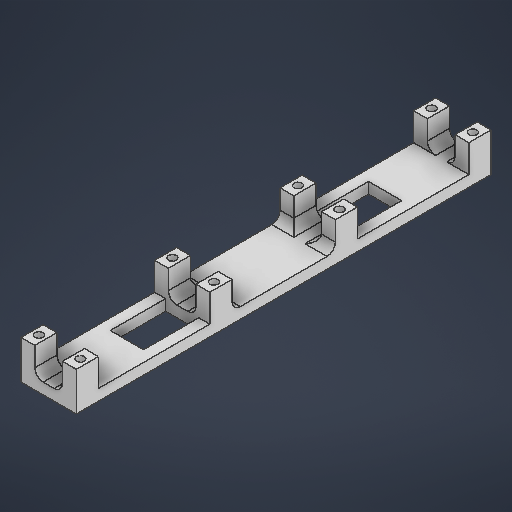
# Autodesk Inventor part: support_2_servos
Saved by Autodesk Inventor 2026.1 (Build 301233000, 233)
## iProperties
Created: 2025-10-11
Part Number: support_2_servos
Material: Generic
Document SubType Name: Modeling
Designer: emanuel
Density: 1 g/cm^3
Appearance: Default
Author: emanuel
Autodesk Inventor part; units mm, degrees
ref_plane "YZ Plane" through (0, 0, 0) normal (1, 0, 0) x (0, 1, 0)
ref_plane "XZ Plane" through (0, 0, 0) normal (0, 1, 0) x (-1, 0, 0)
ref_plane "XY Plane" through (0, 0, 0) normal (0, 0, 1) x (1, 0, 0)
sketch "Sketch1" plane through (0, 0, 0) normal (0, 1, 0) x (-1, 0, 0)
  line L0 (0, 0) -> (20, 0)
  line L1 (20, 0) -> (20, -150)
  line L2 (20, -150) -> (0, -150)
  line L3 (0, -150) -> (0, 0)
  dimension "d0" = 20
  dimension "d1" = 150
  constraints: 8 end point, 2 parallel, 1 horizontal, 1 perpendicular
  measures "d0" distance of L1.end L2.end
  measures "d1" distance of L0.end L1.end
extrude "Extrusion1" add sketch "Sketch1" along normal blind 4
sketch "Sketch2" plane through (0, 4, 0) normal (0, 1, 0) x (1, 0, 0)
  line L0 (-20, 0) -> (0, 0) projected
  line L1 (0, 0) -> (0, 150) projected
  line L2 (-20, 0) -> (0, 0)
  line L3 (0, 0) -> (0, 8)
  line L4 (0, 8) -> (-20, 8)
  line L5 (-20, 8) -> (-20, 0)
  line L6 (-20, 8) -> (0, 8)
  line L7 (0, 8) -> (0, 48.3)
  line L8 (0, 48.3) -> (-20, 48.3)
  line L9 (-20, 48.3) -> (-20, 8)
  line L10 (-20, 48.3) -> (0, 48.3)
  line L11 (0, 48.3) -> (0, 56.3)
  line L12 (0, 56.3) -> (-20, 56.3)
  line L13 (-20, 56.3) -> (-20, 48.3)
  line L14 (-20, 150) -> (-20, 0) projected
  line L15 (-20, 150) -> (0, 150)
  line L16 (0, 150) -> (0, 142)
  line L17 (0, 142) -> (-20, 142)
  line L18 (-20, 142) -> (-20, 150)
  line L19 (-20, 142) -> (0, 142)
  line L20 (0, 142) -> (0, 101.7)
  line L21 (0, 101.7) -> (-20, 101.7)
  line L22 (-20, 101.7) -> (-20, 142)
  line L23 (-20, 101.7) -> (0, 101.7)
  line L24 (0, 101.7) -> (0, 93.7)
  line L25 (0, 93.7) -> (-20, 93.7)
  line L26 (-20, 93.7) -> (-20, 101.7)
  line L27 (-20, 0) -> (-15, 0)
  line L28 (-15, 0) -> (-15, 8)
  line L29 (-15, 8) -> (-20, 8)
  line L30 (-20, 8) -> (-20, 0)
  line L31 (0, 8) -> (-5, 8)
  line L32 (-5, 8) -> (-5, 0)
  line L33 (-5, 0) -> (0, 0)
  line L34 (0, 0) -> (0, 8)
  line L35 (-20, 48.3) -> (-15, 48.3)
  line L36 (-15, 48.3) -> (-15, 56.3)
  line L37 (-15, 56.3) -> (-20, 56.3)
  line L38 (-20, 56.3) -> (-20, 48.3)
  line L39 (0, 48.3) -> (-5, 48.3)
  line L40 (-5, 48.3) -> (-5, 56.3)
  line L41 (-5, 56.3) -> (0, 56.3)
  line L42 (0, 56.3) -> (0, 48.3)
  line L43 (-20, 93.7) -> (-15, 93.7)
  line L44 (-15, 93.7) -> (-15, 101.7)
  line L45 (-15, 101.7) -> (-20, 101.7)
  line L46 (-20, 101.7) -> (-20, 93.7)
  line L47 (0, 93.7) -> (-5, 93.7)
  line L48 (-5, 93.7) -> (-5, 101.7)
  line L49 (-5, 101.7) -> (0, 101.7)
  line L50 (0, 101.7) -> (0, 93.7)
  line L51 (-20, 142) -> (-15, 142)
  line L52 (-15, 142) -> (-15, 150)
  line L53 (-15, 150) -> (-20, 150)
  line L54 (-20, 150) -> (-20, 142)
  line L55 (0, 142) -> (-5, 142)
  line L56 (-5, 142) -> (-5, 150)
  line L57 (-5, 150) -> (0, 150)
  line L58 (0, 150) -> (0, 142)
  point P0 (0, 142)
  point P1 (-20, 142)
  point P2 (-15, 93.7)
  point P3 (-15, 101.7)
  point P4 (-20, 101.7)
  point P5 (-20, 93.7)
  dimension "d4" = 8
  dimension "d5" = 40.3
  dimension "d6" = 8
  dimension "d7" = 20
  dimension "d8" = 8
  dimension "d9" = 40.3
  dimension "d10" = 8
  dimension "d11" = 5
  dimension "d12" = 5
  dimension "d13" = 8
  dimension "d14" = 5
  dimension "d15" = 5
  dimension "d16" = 5
  dimension "d17" = 5
  dimension "d18" = 5
  dimension "d19" = 5
  constraints: 112 end point, 28 parallel, 14 horizontal, 14 perpendicular, 12 point on line
  measures "d4" distance of L3.end L2.end
  measures "d5" distance of L7.end L6.end
  measures "d6" distance of L11.end L10.end
  measures "d7" distance of L16.end L17.end
  measures "d8" distance of L15.end L16.end
  measures "d9" distance of L19.end L20.end
  measures "d10" distance of L23.end L24.end
  measures "d11" distance of L29.end L28.end
  measures "d12" distance of L33.end L32.end
  measures "d13" distance of L32.end L31.end
  measures "d14" distance of L37.end L36.end
  measures "d15" distance of L40.end L41.end
  measures "d16" distance of L45.end L44.end
  measures "d17" distance of L48.end L49.end
  measures "d18" distance of L53.end L52.end
  measures "d19" distance of L56.end L57.end
extrude "Extrusion2" add sketch "Sketch2" along normal blind 10 contours L5 L4 L28 L0 | L32 L4 L1 L0 | L13 L12 L36 L8 | L40 L12 L1 L8 | L14 L21 L44 L25 | L14 L15 L52 L17 | L48 L21 L1 L25 | L56 L15 L1 L17
sketch "Sketch3" plane through (0, 14, 0) normal (0, 1, 0) x (1, 0, 0)
  line L0 (-20, 150) -> (-20, 0) projected
  line L1 (-20, 0) -> (-17.5, 0)
  line L2 (-17.5, 0) -> (-17.5, 4)
  line L3 (-17.5, 4) -> (-20, 4)
  line L4 (-20, 4) -> (-20, 0)
  line L5 (0, 0) -> (0, 150) projected
  line L6 (0, 0) -> (-2.5, 0)
  line L7 (-2.5, 0) -> (-2.5, 4)
  line L8 (-2.5, 4) -> (0, 4)
  line L9 (0, 4) -> (0, 0)
  line L10 (-15, 56.3) -> (-20, 56.3) projected
  line L11 (-20, 56.3) -> (-17.5, 56.3)
  line L12 (-17.5, 56.3) -> (-17.5, 52.3)
  line L13 (-17.5, 52.3) -> (-20, 52.3)
  line L14 (-20, 52.3) -> (-20, 56.3)
  line L15 (-5, 56.3) -> (0, 56.3) projected
  line L16 (-5, 56.3) -> (-2.5, 56.3)
  line L17 (-2.5, 56.3) -> (-2.5, 52.3)
  line L18 (-2.5, 52.3) -> (-5, 52.3)
  line L19 (-5, 52.3) -> (-5, 56.3)
  line L20 (-20, 150) -> (-17.5, 150)
  line L21 (-17.5, 150) -> (-17.5, 146)
  line L22 (-17.5, 146) -> (-20, 146)
  line L23 (-20, 146) -> (-20, 150)
  line L24 (-5, 150) -> (-2.5, 150)
  line L25 (-2.5, 150) -> (-2.5, 146)
  line L26 (-2.5, 146) -> (-5, 146)
  line L27 (-5, 146) -> (-5, 150)
  line L28 (-20, 101.7) -> (-15, 101.7) projected
  line L29 (-15, 101.7) -> (-17.5, 101.7)
  line L30 (-17.5, 101.7) -> (-17.5, 97.7)
  line L31 (-17.5, 97.7) -> (-15, 97.7)
  line L32 (-15, 97.7) -> (-15, 101.7)
  line L33 (-5, 101.7) -> (-2.5, 101.7)
  line L34 (-2.5, 101.7) -> (-2.5, 97.7)
  line L35 (-2.5, 97.7) -> (-5, 97.7)
  line L36 (-5, 97.7) -> (-5, 101.7)
  circle A0 centre (-17.5, 97.7) radius 1.5
  circle A1 centre (-2.5, 97.7) radius 1.5
  circle A2 centre (-17.5, 146) radius 1.5
  circle A3 centre (-2.5, 146) radius 1.5
  circle A4 centre (-17.5, 52.3) radius 1.5
  circle A5 centre (-2.5, 52.3) radius 1.5
  circle A6 centre (-17.5, 4) radius 1.5
  circle A7 centre (-2.5, 4) radius 1.5
  dimension "d22" = 2.5
  dimension "d23" = 4
  dimension "d24" = 2.5
  dimension "d25" = 4
  dimension "d26" = 2.5
  dimension "d27" = 4
  dimension "d28" = 2.5
  dimension "d29" = 4
  dimension "d30" = 2.5
  dimension "d31" = 4
  dimension "d32" = 2.5
  dimension "d33" = 4
  dimension "d34" = 2.5
  dimension "d35" = 4
  dimension "d36" = 2.5
  dimension "d37" = 4
  dimension "d38" = 3
  dimension "d39" = 3
  dimension "d40" = 3
  dimension "d41" = 3
  dimension "d42" = 3
  dimension "d43" = 3
  dimension "d44" = 3
  dimension "d45" = 3
  constraints: 64 end point, 16 parallel, 8 centre point, 8 coincident, 8 horizontal, 8 perpendicular, 4 point on line
  measures "d22" distance of L3.end L2.end
  measures "d23" distance of L2.end L1.end
  measures "d24" distance of L7.end L8.end
  measures "d25" distance of L6.end L7.end
  measures "d26" distance of L12.end L13.end
  measures "d27" distance of L11.end L12.end
  measures "d28" distance of L17.end L18.end
  measures "d29" distance of L16.end L17.end
  measures "d30" distance of L21.end L22.end
  measures "d31" distance of L20.end L21.end
  measures "d32" distance of L25.end L26.end
  measures "d33" distance of L24.end L25.end
  measures "d34" distance of L31.end L30.end
  measures "d35" distance of L30.end L29.end
  measures "d36" distance of L34.end L35.end
  measures "d37" distance of L33.end L34.end
  measures "d38" diameter of A0
  measures "d39" diameter of A1
  measures "d40" diameter of A2
  measures "d41" diameter of A3
  measures "d42" diameter of A4
  measures "d43" diameter of A5
  measures "d44" diameter of A6
  measures "d45" diameter of A7
extrude "Extrusion3" cut sketch "Sketch3" against normal up to surface (14 mm away) contours A2 L21 L22 | L22 L21 A2 | A4 L12 L13 | L13 L12 A4 | A6 L2 L3 | L3 L2 A6 | A7 L7 L8 | L8 L7 A7 | A5 L18 L17 | L17 L18 A5 | A3 L26 L25 | L25 L26 A3 | A0 L31 L30 | L30 L31 A0 | A1 L35 L34 | L34 L35 A1
fillet "Fillet1" radius 3 12 edges at (-15, 4, -52.3) (-5, 4, -52.3) (-15, 4, -97.7) (-17.5, 4, -93.7) (-17.5, 4, -56.3) (-2.5, 4, -93.7) (-2.5, 4, -56.3) (-5, 4, -97.7) (-15, 4, -4) (-5, 4, -4) (-15, 4, -146) (-5, 4, -146)
sketch "Sketch5" plane through (0, 4, 0) normal (0, 1, 0) x (1, 0, 0)
  line L0 (0, 48.3) -> (-8, 48.3) projected
  line L1 (0, 48.3) -> (-4, 48.3)
  line L2 (-8, 101.7) -> (0, 101.7) projected
  line L3 (0, 101.7) -> (-4, 101.7)
  line L4 (-4, 101.7) -> (-16, 101.7)
  line L5 (-16, 101.7) -> (-16, 121.7)
  line L6 (-16, 121.7) -> (-4, 121.7)
  line L7 (-4, 121.7) -> (-4, 101.7)
  line L8 (-4, 48.3) -> (-16, 48.3)
  line L9 (-16, 48.3) -> (-16, 28.3)
  line L10 (-16, 28.3) -> (-4, 28.3)
  line L11 (-4, 28.3) -> (-4, 48.3)
  point P0 (0, 0)
  dimension "d63" = 4
  dimension "d64" = 4
  dimension "d65" = 12
  dimension "d66" = 20
  dimension "d67" = 12
  dimension "d68" = 20
  constraints: 20 end point, 4 parallel, 2 horizontal, 2 midpoint, 2 perpendicular
  measures "d63" distance of L0.start L1.end
  measures "d64" distance of L2.end L3.end
  measures "d65" distance of L5.end L6.end
  measures "d66" distance of L4.end L5.end
  measures "d67" distance of L10.end L9.end
  measures "d68" distance of L9.end L8.end
extrude "Extrusion5" cut sketch "Sketch5" against normal blind 8
sketch "Sketch6" plane through (0, 0, 0) normal (0, -1, 0) x (1, 0, 0)
  circle A0 centre (-2.5, -4) radius 1.5 projected
  circle A1 centre (-2.5, -4) radius 4
  circle A2 centre (-17.5, -4) radius 1.5 projected
  circle A3 centre (-17.5, -4) radius 4
  circle A4 centre (-17.5, -52.3) radius 1.5 projected
  circle A5 centre (-17.5, -52.3) radius 4
  circle A6 centre (-2.5, -52.3) radius 1.5 projected
  circle A7 centre (-2.5, -52.3) radius 4
  circle A8 centre (-17.5, -97.7) radius 1.5 projected
  circle A9 centre (-17.5, -97.7) radius 4
  circle A10 centre (-2.5, -97.7) radius 1.5 projected
  circle A11 centre (-2.5, -97.7) radius 4
  circle A12 centre (-17.5, -146) radius 1.5 projected
  circle A13 centre (-17.5, -146) radius 4
  circle A14 centre (-2.5, -146) radius 1.5 projected
  circle A15 centre (-2.5, -146) radius 4
  line L0 (0, -150) -> (-20, -150) projected
  line L1 (-20, -150) -> (-17.5, -150)
  line L2 (-17.5, -150) -> (-17.5, -146)
  line L3 (-17.5, -146) -> (-20, -146)
  line L4 (-20, -146) -> (-20, -150)
  line L5 (0, -150) -> (-2.5, -150)
  line L6 (-2.5, -150) -> (-2.5, -146)
  line L7 (-2.5, -146) -> (0, -146)
  line L8 (0, -146) -> (0, -150)
  line L9 (-20, -150) -> (-20, 0) projected
  line L10 (-20, 0) -> (-17.5, 0)
  line L11 (-17.5, 0) -> (-17.5, -4)
  line L12 (-17.5, -4) -> (-20, -4)
  line L13 (-20, -4) -> (-20, 0)
  line L14 (0, 0) -> (-2.5, 0)
  line L15 (-2.5, 0) -> (-2.5, -4)
  line L16 (-2.5, -4) -> (0, -4)
  line L17 (0, -4) -> (0, 0)
  dimension "d71" = 8
  dimension "d72" = 8
  dimension "d73" = 8
  dimension "d74" = 8
  dimension "d75" = 8
  dimension "d76" = 8
  dimension "d77" = 8
  constraints: 32 end point, 8 centre point, 8 coincident, 8 parallel, 4 horizontal, 4 perpendicular, 1 tangent
  measures "d71" diameter of A1
  measures "d72" diameter of A3
  measures "d73" diameter of A5
  measures "d74" diameter of A7
  measures "d75" diameter of A9
  measures "d76" diameter of A11
  measures "d77" diameter of A13
body "Solid1"
